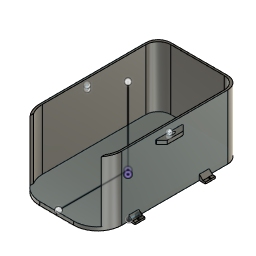
Drone_BatteryHolder v3 (Autodesk Fusion 360 design; units mm, degrees)
Autodesk Fusion 360 part; units mm, degrees
note: some values were not read from the file. Chosen so that the rebuilt part matches the saved one: which face or edge a step refers to; how an offset face is resized; which pieces of a blend or face edit are solid.
sketch "Sketch1" plane through (0, 0, 0) normal (0, 0, 1) x (1, 0, 0)
sketch "Sketch2" plane through (0, 0, 0) normal (0, 0, 1) x (1, 0, 0)
sketch "Sketch3" plane through (0, 0, 0) normal (0, 0, 1) x (1, 0, 0)
sketch "Sketch4" plane through (0, 0, 0) normal (0, 0, 1) x (1, 0, 0)
sketch "Sketch5" plane through (0, 0, 0) normal (0, 0, 1) x (1, 0, 0)
sketch "Sketch6" plane through (0, 0, 0) normal (0, 0, 1) x (1, 0, 0)
sketch "Sketch7" plane through (0, 0, 0) normal (0, 0, 1) x (1, 0, 0)
sketch "Sketch8" plane through (0, 0, 0) normal (0, 0, 1) x (1, 0, 0)
sketch "Sketch9" plane through (0, 0, 0) normal (0, 0, 1) x (1, 0, 0)
sketch "Sketch10" plane through (0, 0, 0) normal (0, 0, 1) x (1, 0, 0)
  line L0 (0, 0) -> (0, 40)
  line L1 (0, 0) -> (23, 0)
  line L2 (0, 0) -> (50, 0) construction
  line L3 (23, 0) -> (23, 40)
  line L4 (23, 40) -> (0, 40)
  line L5 (23, -40) -> (0, -40)
  line L6 (23, 0) -> (23, -40)
  line L7 (0, 0) -> (0, -40)
  line L8 (-23, 40) -> (0, 40)
  line L9 (-23, 0) -> (-23, 40)
  line L10 (0, 0) -> (-50, 0) construction
  line L11 (-23, 0) -> (-23, -40)
  line L12 (-23, -40) -> (0, -40)
  line L13 (0, 0) -> (-23, 0)
  dimension "d15" = 40
  dimension "d16" = 23
  constraint coincident L0.start L1.start
  constraint vertical L0
  constraint perpendicular L0 L1
  constraint horizontal L2
  constraint perpendicular L1 L3
  constraint symmetric L0.start L1 L2.start
  constraint symmetric L0.end L1 L5.end
  constraint symmetric L3.start L1 L6.start
  constraint symmetric L1 L3.end L5.start
  constraint symmetric L4.end L0 L8.end
  constraint symmetric L0 L1.end L9.start
  constraint symmetric L0 L1.start L2.start
  constraint symmetric L0 L2.end L10.end
  constraint symmetric L0 L3.end L8.start
  constraint symmetric L0.start L7 L1.start
  constraint symmetric L1.end L7 L9.start
  constraint symmetric L5.start L7 L11.end
  constraint symmetric L5.end L7 L12.end
  measures "d15" distance of L0.start L0.end
  measures "d16" distance of L0.start L1.end
extrude "Extrude1" add sketch "Sketch10" along normal blind 2
fillet "Fillet1" radius 7 2 edges at (23, 40, 1) (-23, 40, 1)
fillet "Fillet2" radius 13.5 2 edges at (-23, -40, 1) (23, -40, 1)
sketch "Sketch11" plane through (0, 0, 2) normal (0, 0, 1) x (-1, 0, 0)
  arc A0 (-9.5, 40) -> (-23, 26.5) centre (-9.5, 26.5) ccw
  line L0 (-23, 26.5) -> (-23, -33)
  arc A1 (-23, -33) -> (-16, -40) centre (-16, -33) ccw
  line L1 (-16, -40) -> (0, -40)
  line L2 (0, -40) -> (16, -40)
  arc A2 (16, -40) -> (23, -33) centre (16, -33) ccw
  line L3 (23, -33) -> (23, 26.5)
  arc A3 (23, 26.5) -> (9.5, 40) centre (9.5, 26.5) ccw
  line L4 (9.5, 40) -> (0, 40)
  line L5 (0, 40) -> (-9.5, 40)
  line L6 (0, 0) -> (0, -40)
  line L7 (0, 0) -> (-23, 0)
  line L8 (-23, 0) -> (-23, -33)
  line L9 (0, -40) -> (-16, -40)
  arc A4 (-23, -33) -> (-16, -40) centre (-16, -33) ccw
  line L10 (0, -39) -> (-15, -39)
  line L11 (-22, 0) -> (-22, -32)
  arc A5 (-22, -32) -> (-15, -39) centre (-15, -32) ccw
  line L12 (0, -39) -> (15, -39)
  line L13 (0, -40) -> (16, -40)
  arc A6 (16, -40) -> (23, -33) centre (16, -33) ccw
  arc A7 (15, -39) -> (22, -32) centre (15, -32) ccw
  line L14 (22, 0) -> (22, -32)
  line L15 (23, 0) -> (23, -33)
  line L16 (0, 0) -> (23, 0)
  line L17 (0, 0) -> (0, 40)
  line L18 (23, 0) -> (23, 26.5)
  line L19 (22, 0) -> (22, 26.0718)
  arc A8 (22, 26.0718) -> (20, 33) centre (9, 26.0718) ccw
  arc A9 (23, 26.5) -> (20.0018, 34.983) centre (9.5, 26.5) ccw
  line L20 (-23, 0) -> (-23, 26.5)
  line L21 (-22, 0) -> (-22, 26.0718)
  arc A10 (-20.0018, 34.983) -> (-23, 26.5) centre (-9.5, 26.5) ccw
  arc A11 (-20, 33) -> (-22, 26.0718) centre (-9, 26.0718) ccw
  line L22 (20.0018, 32.9971) -> (20.0018, 34.983)
  line L23 (-20.0018, 32.9971) -> (-20.0018, 34.983)
  dimension "d25" = 7
  dimension "d26" = 7
  constraint coincident L6.start L7.start
  constraint coincident L1.end L2.start
  constraint coincident L0 L7.end
  constraint perpendicular L0 L7
  constraint tangent L9 A4
  constraint tangent L8 A4
  constraint coincident L6 L10.start
  constraint perpendicular L6 L10
  constraint coincident L7 L11.start
  constraint perpendicular L7 L11
  constraint tangent L11 A5
  constraint tangent L10 A5
  constraint symmetric L1.end L6 L2.start
  constraint symmetric L6 L7.end L15.start
  constraint symmetric L6 A1.end L2.end
  constraint symmetric L6 L0.end A2.end
  constraint symmetric L6 A4 A6
  constraint symmetric L6 L10.start L12.start
  constraint symmetric L6 L11.start L14.start
  constraint symmetric L6 L11.end A7.end
  constraint symmetric L6 L10.end L12.end
  constraint symmetric L6 A5 A7
  constraint perpendicular L15 L16
  constraint coincident L4.end L5.start
  constraint parallel L3 L18
  constraint parallel L18 L19
  constraint tangent L19 A8
  constraint tangent L18 A9
  constraint symmetric L14.start L17 L11.start
  constraint symmetric L15.start L17 L7.end
  constraint symmetric L17 L19.end L21.end
  constraint symmetric L17 A8.end A11.start
  constraint symmetric L17 A8 A11
  constraint symmetric L17 L3.end A0.end
  constraint symmetric L17 A10.start A9.end
  constraint symmetric L17 A9 A10
  constraint coincident A8 L22.start
  constraint coincident A9 L22.end
  constraint vertical L22
  constraint symmetric L17 L22.start L23.start
  constraint symmetric L17 A9.end A10.start
  constraint coincident A0 A10.start
  measures "d25" radius of A4
  measures "d26" radius of A5
extrude "Extrude2" add sketch "Sketch11" along normal blind 34 contours A0 L0 L7 L20 L21 A10 A11 L23 | L0 A1 L1 L6 L7 L8 L9 A4 L10 L11 A5 | L3 A3 L16 L18 L19 A8 A9 L22 | L2 A2 L3 L6 L12 L13 A6 A7 L14 L15 L16
sketch "Sketch12" plane through (0, 0, 0) normal (0, 1, 0) x (1, 0, 0)
  line L0 (23, -30) -> (23, -32)
  line L1 (-23, -30) -> (-23, -32)
  constraint vertical L0
sketch "Sketch13" plane through (23, 0, 0) normal (1, 0, 0) x (0, 1, 0)
  line L0 (-26.5, 36) -> (-26.5, 0)
  line L1 (-26.5, 0) -> (33, 0)
  line L2 (33, 0) -> (33, 36)
  line L3 (33, 36) -> (-26.5, 36)
  line L4 (0, 50) -> (0, 0)
  line L5 (0, 32) -> (7.5, 32)
  line L6 (0, 32) -> (-7.5, 32)
  line L7 (7.5, 32) -> (7.5, 30)
  line L8 (7.5, 30) -> (0, 30)
  line L9 (-7.5, 32) -> (-7.5, 30)
  line L10 (-7.5, 30) -> (0, 30)
  dimension "d31" = 7.5
  constraint coincident L4.end origin
  constraint perpendicular L1 L4
  constraint coincident L4 L5.start
  constraint perpendicular L4 L5
  constraint symmetric L4 L5.start L6.start
  constraint symmetric L4 L5.end L6.end
  constraint perpendicular L5 L7
  constraint coincident L4 L8.end
  constraint perpendicular L4 L8
  constraint symmetric L4 L7.end L9.end
  constraint symmetric L4 L8.end L10.end
  measures "d31" distance of L5.start L5.end
sketch "Sketch14" plane through (-23, 0, 0) normal (-1, 0, 0) x (0, -1, 0)
  line L0 (26.5, 0) -> (26.5, 36)
  line L1 (26.5, 36) -> (-33, 36)
  line L2 (-33, 36) -> (-33, 0)
  line L3 (-33, 0) -> (26.5, 0)
  line L4 (0, 32) -> (7.5, 32)
  line L5 (7.5, 32) -> (7.5, 30)
  line L6 (7.5, 30) -> (0, 30)
  line L7 (0, 45) -> (0, 0)
  line L8 (0, 0) -> (44, 0)
  line L9 (0, 32) -> (-7.5, 32)
  line L10 (-7.5, 32) -> (-7.5, 30)
  line L11 (-7.5, 30) -> (0, 30)
  dimension "d32" = 7.5
  constraint parallel L1 L4
  constraint perpendicular L1 L5
  constraint perpendicular L5 L6
  constraint coincident L7.end L8.start
  constraint perpendicular L3 L7
  constraint perpendicular L7 L8
  constraint symmetric L4.start L7 L9.start
  constraint symmetric L4.end L7 L9.end
  constraint symmetric L5.end L7 L10.end
  constraint symmetric L6.end L7 L11.end
  measures "d32" distance of L4.start L4.end
sketch "Sketch15" plane through (0, 0, 0) normal (0, 1, 0) x (1, 0, 0)
  line L0 (0, 0) -> (0, -45)
  constraint coincident L0.start origin
  constraint vertical L0
extrude "Extrude3" add sketch "Sketch14" along normal blind 3.5 contours L4 L5 L6 L7 | L7 L9 L10 L11
extrude "Extrude4" add sketch "Sketch13" along normal blind 3.5 contours L4 L5 L7 L8 | L4 L6 L9 L10
sketch "Sketch16" plane through (0, 0, 2) normal (0, 0, 1) x (-1, 0, 0)
  line L0 (20.0018, 32.9971) -> (20.0018, 34.983)
  arc A0 (20.0018, 34.983) -> (9.5, 40) centre (9.5, 26.5) ccw
  line L1 (9.5, 40) -> (0, 40)
  line L2 (0, 40) -> (-9.5, 40)
  arc A1 (-9.5, 40) -> (-20.0018, 34.983) centre (-9.5, 26.5) ccw
  line L3 (-20.0018, 34.983) -> (-20.0018, 32.9971)
  arc A2 (-20.0018, 32.9971) -> (-22, 26.0718) centre (-9, 26.0718) ccw
  line L4 (-22, 26.0718) -> (-22, -32)
  arc A3 (-22, -32) -> (-15, -39) centre (-15, -32) ccw
  line L5 (-15, -39) -> (15, -39)
  arc A4 (15, -39) -> (22, -32) centre (15, -32) ccw
  line L6 (22, -32) -> (22, 26.0718)
  arc A5 (22, 26.0718) -> (20.0018, 32.9971) centre (9, 26.0718) ccw
chamfer "Chamfer1" distance 3 angle 45 2 edges at (-26.5, 7.5, 31) (-26.5, -7.5, 31)
chamfer "Chamfer2" distance 3 angle 45 2 edges at (26.5, 7.5, 31) (26.5, -7.5, 31)
sketch "Sketch17" plane through (0, 0, 2) normal (0, 0, 1) x (-1, 0, 0)
sketch "Sketch18" plane through (0, 0, 32) normal (0, 0, 1) x (-1, 0, 0)
  line L0 (26.5, 4.5) -> (23.5, 7.5)
  line L1 (23.5, 7.5) -> (23, 7.5)
  line L2 (23, 7.5) -> (23, -7.5)
  line L3 (23, -7.5) -> (23.5, -7.5)
  line L4 (23.5, -7.5) -> (26.5, -4.5)
  line L5 (26.5, -4.5) -> (26.5, 4.5)
  line L6 (0, 0) -> (0, -49)
  ellipse E0 centre (24.5, 0) end of major axis (24.5, -2) minor radius 0.75
  line L7 (24.5, 2) -> (24.5, -2)
  line L8 (23.75, 0) -> (25.25, 0)
  dimension "d39" = 1.5
  constraint coincident L6.start origin
  constraint vertical L6
  constraint vertical L7
  constraint coincident E0 L7.start
  constraint coincident E0 L7.end
  constraint coincident E0 L8.start
  constraint coincident E0 L8.end
extrude "Extrude5" cut sketch "Sketch18" against normal blind 2 contours E0 L7 L8 | E0 L7 L8 | E0 L7 L8 | E0 L7 L8
sketch "Sketch19" plane through (0, 0, 32) normal (0, 0, 1) x (-1, 0, 0)
  ellipse E0 centre (24.5, 0) end of major axis (24.5, -2) minor radius 0.75
  line L0 (26.5, 4.5) -> (23.5, 7.5)
  line L1 (23.5, 7.5) -> (23, 7.5)
  line L2 (23, 7.5) -> (23, -7.5)
  line L3 (23, -7.5) -> (23.5, -7.5)
  line L4 (23.5, -7.5) -> (26.5, -4.5)
  line L5 (26.5, -4.5) -> (26.5, 4.5)
  line L6 (0, 0) -> (0, -26)
  ellipse E1 centre (-24.5, 0) end of major axis (-24.5, -2) minor radius 0.75
  constraint coincident L6.start origin
  constraint vertical L6
  constraint symmetric E0 L6 E1
extrude "Extrude6" cut sketch "Sketch19" against normal blind 2 contours E1
sketch "Sketch20" plane through (-23, 0, 0) normal (-1, 0, 0) x (0, -1, 0)
  line L0 (7.5, 32) -> (7.5, 30)
  line L1 (7.5, 30) -> (-7.5, 30)
  line L2 (-7.5, 30) -> (-7.5, 32)
  line L3 (-7.5, 32) -> (7.5, 32)
  line L4 (26.5, 0) -> (26.5, 36)
  line L5 (26.5, 36) -> (-33, 36)
  line L6 (-33, 36) -> (-33, 0)
  line L7 (-33, 0) -> (26.5, 0)
  line L8 (0, 45) -> (0, 0)
  line L9 (0, 0) -> (50, 0)
  line L10 (26.5, 0) -> (22.5, 0)
  line L11 (22.5, 0) -> (22.5, 3)
  line L12 (22.5, 3) -> (17, 3)
  line L13 (17, 3) -> (17, 0)
  line L14 (-22.5, 0) -> (-22.5, 3)
  line L15 (-22.5, 3) -> (-17, 3)
  line L16 (-17, 3) -> (-17, 0)
  dimension "d44" = 4
  constraint coincident L8.end L9.start
  constraint perpendicular L7 L8
  constraint perpendicular L8 L9
  constraint coincident L4.start L7.end
  constraint perpendicular L4 L10
  constraint perpendicular L9 L11
  constraint perpendicular L11 L12
  constraint coincident L9 L13.end
  constraint perpendicular L12 L13
  constraint symmetric L8 L10.end L14.start
  constraint symmetric L8 L11.end L14.end
  constraint symmetric L8 L12.end L15.end
  constraint symmetric L8 L13.end L16.end
  measures "d44" distance of L4.start L10.end
extrude "Extrude7" add sketch "Sketch20" along normal blind 2 contours L7 L14 L15 L16 | L7 L9 L11 L12 L13
sketch "Sketch21" plane through (-23, 0, 0) normal (-1, 0, 0) x (0, -1, 0)
  line L0 (22.5, 3) -> (22.5, 0)
  line L1 (22.5, 0) -> (26.5, 0)
  line L2 (26.5, 0) -> (26.5, 36)
  line L3 (26.5, 36) -> (-33, 36)
  line L4 (-33, 36) -> (-33, 0)
  line L5 (-33, 0) -> (-22.5, 0)
  line L6 (-22.5, 0) -> (-22.5, 3)
  line L7 (-22.5, 3) -> (-17, 3)
  line L8 (-17, 3) -> (-17, 0)
  line L9 (-17, 0) -> (17, 0)
  line L10 (17, 0) -> (17, 3)
  line L11 (17, 3) -> (22.5, 3)
  line L12 (7.5, 32) -> (7.5, 30)
  line L13 (7.5, 30) -> (-7.5, 30)
  line L14 (-7.5, 30) -> (-7.5, 32)
  line L15 (-7.5, 32) -> (7.5, 32)
sketch "Sketch22" plane through (23, 0, 0) normal (1, 0, 0) x (0, 1, 0)
  line L0 (7.5, 32) -> (7.5, 30)
  line L1 (7.5, 30) -> (-7.5, 30)
  line L2 (-7.5, 30) -> (-7.5, 32)
  line L3 (-7.5, 32) -> (7.5, 32)
  line L4 (-26.5, 36) -> (-26.5, 0)
  line L5 (-26.5, 0) -> (33, 0)
  line L6 (33, 0) -> (33, 36)
  line L7 (33, 36) -> (-26.5, 36)
  line L8 (0, 45) -> (0, 0)
  line L9 (0, 0) -> (50, 0)
  line L10 (-26.5, 0) -> (-22.5, 0)
  line L11 (-22.5, 0) -> (-22.5, 3)
  line L12 (-22.5, 3) -> (-18.5, 3)
  line L13 (-18.5, 3) -> (-18.5, 0)
  line L14 (22.5, 0) -> (22.5, 3)
  line L15 (22.5, 3) -> (18.5, 3)
  line L16 (18.5, 3) -> (18.5, 0)
  dimension "d47" = 4
  dimension "d48" = 3
  dimension "d49" = 4
  constraint coincident L8.end L9.start
  constraint perpendicular L5 L8
  constraint perpendicular L8 L9
  constraint coincident L4.end L5.start
  constraint perpendicular L4 L10
  constraint perpendicular L10 L11
  constraint perpendicular L11 L12
  constraint coincident L5 L13.end
  constraint perpendicular L5 L13
  constraint symmetric L8 L10.end L14.start
  constraint symmetric L8 L11.end L14.end
  constraint symmetric L8 L12.end L15.end
  constraint symmetric L8 L13.end L16.end
  measures "d47" distance of L4.end L10.end
  measures "d48" distance of L10.end L11.end
  measures "d49" distance of L11.end L12.end
extrude "Extrude8" add sketch "Sketch22" along normal blind 2 contours L5 L11 L12 L13 | L5 L9 L14 L15 L16
delete_face "DeleteFace1" 5 faces at (24.3333, -22.5, 1.6667) (23.6667, -21.1667, 3) (24.3333, -18.5, 1.6667) (23.6667, -21.1667, 0) (25, -19.8333, 1)
delete_face "DeleteFace2" 1 faces at (23.6667, 21.1667, 3)
sketch "Sketch23" plane through (23, 0, 0) normal (1, 0, 0) x (0, 1, 0)
  line L0 (7.5, 32) -> (7.5, 30)
  line L1 (7.5, 30) -> (-7.5, 30)
  line L2 (-7.5, 30) -> (-7.5, 32)
  line L3 (-7.5, 32) -> (7.5, 32)
  line L4 (33, 36) -> (-26.5, 36)
  line L5 (-26.5, 36) -> (-26.5, 0)
  line L6 (-26.5, 0) -> (33, 0)
  line L7 (33, 0) -> (33, 36)
  line L8 (0, 0) -> (0, 45)
  line L9 (0, 0) -> (45, 0)
  line L10 (-26.5, 0) -> (-22.5, 0)
  line L11 (-22.5, 0) -> (-17, 0)
  line L12 (-22.5, 0) -> (-22.5, 3)
  line L13 (-22.5, 3) -> (-17, 3)
  line L14 (-17, 3) -> (-17, 0)
  line L15 (22.5, 0) -> (22.5, 3)
  line L16 (22.5, 3) -> (17, 3)
  line L17 (17, 3) -> (17, 0)
  dimension "d52" = 4
  constraint coincident L8.start L9.start
  constraint perpendicular L4 L8
  constraint perpendicular L8 L9
  constraint coincident L5.end L6.start
  constraint coincident L6 L10.end
  constraint coincident L6 L11.end
  constraint perpendicular L11 L12
  constraint perpendicular L12 L13
  constraint perpendicular L6 L14
  constraint symmetric L8 L10.end L15.start
  constraint symmetric L8 L11.end L17.end
  constraint symmetric L8 L12.end L15.end
  constraint symmetric L8 L13.end L16.end
  measures "d52" distance of L5.end L10.end
extrude "Extrude9" add sketch "Sketch23" along normal blind 2 contours L6 L11 L12 L13 L14 | L6 L9 L15 L16 L17
chamfer "Chamfer3" distance 2 angle 45 4 edges at (25, -19.75, 3) (25, 19.75, 3) (-25, -19.75, 3) (-25, 19.75, 3)
sketch "Sketch24" plane through (23, 0, 0) normal (1, 0, 0) x (0, 1, 0)
  line L0 (22.5, 3) -> (22.5, 0)
  line L1 (22.5, 0) -> (33, 0)
  line L2 (33, 0) -> (33, 36)
  line L3 (33, 36) -> (-26.5, 36)
  line L4 (-26.5, 36) -> (-26.5, 0)
  line L5 (-26.5, 0) -> (-22.5, 0)
  line L6 (-22.5, 0) -> (-22.5, 3)
  line L7 (-22.5, 3) -> (-17, 3)
  line L8 (-17, 3) -> (-17, 0)
  line L9 (-17, 0) -> (17, 0)
  line L10 (17, 0) -> (17, 3)
  line L11 (17, 3) -> (22.5, 3)
  line L12 (7.5, 32) -> (7.5, 30)
  line L13 (7.5, 30) -> (-7.5, 30)
  line L14 (-7.5, 30) -> (-7.5, 32)
  line L15 (-7.5, 32) -> (7.5, 32)
  line L16 (-22.5, 0.9094) -> (-17, 0.9094)
  line L17 (-17, 0.9094) -> (-17, 0)
  line L18 (-17, 0) -> (-22.5, 0)
  line L19 (-22.5, 0) -> (-22.5, 0.9094)
  constraint horizontal L16
  constraint vertical L17
  constraint horizontal L18
  constraint vertical L19
  constraint coincident L8.end L9.start
  constraint coincident L6 L16.start
sketch "Sketch25" plane through (0, 0, 2) normal (0, 0, 1) x (-1, 0, 0)
sketch "Sketch26" plane through (0, 0, 2) normal (0, 0, 1) x (-1, 0, 0)
sketch "Sketch27" plane through (0, 0, 2) normal (0, 0, 1) x (-1, 0, 0)
sketch "Sketch28" plane through (0, 0, 0) normal (0, 0, 1) x (1, 0, 0)
sketch "Sketch29" plane through (0, 0, 0) normal (0, 0, 1) x (1, 0, 0)
sketch "Sketch30" plane through (0, 0, 0) normal (0, 0, 1) x (1, 0, 0)
  line L0 (0, -50) -> (0, 45)
  line L1 (-35, 0) -> (39, 0)
  line L2 (-25, -22.5) -> (-26.5, -22.5)
  line L3 (-26.5, -22.5) -> (-26.5, -17)
  line L4 (-26.5, -17) -> (-25, -17)
  line L5 (-25, -17) -> (-25, -22.5)
  line L6 (-26.5, 22.5) -> (-26.5, 17)
  line L7 (-25, 22.5) -> (-26.5, 22.5)
  line L8 (-25, 17) -> (-25, 22.5)
  line L9 (-26.5, 17) -> (-25, 17)
  constraint vertical L0
  constraint horizontal L1
  constraint horizontal L2
  constraint vertical L3
  constraint horizontal L4
  constraint vertical L5
  constraint symmetric L1 L2.start L7.start
  constraint symmetric L1 L2.end L6.start
  constraint symmetric L1 L3.end L6.end
  constraint symmetric L1 L4.end L8.start
extrude "Extrude10" add sketch "Sketch30" along normal blind 1
sketch "Sketch31" plane through (0, 0, 0) normal (0, 0, 1) x (1, 0, 0)
  line L0 (0, 0) -> (40, 0)
  line L1 (25, -22.5) -> (26.5, -22.5)
  line L2 (26.5, -22.5) -> (26.5, -17)
  line L3 (26.5, -17) -> (25, -17)
  line L4 (25, -17) -> (25, -22.5)
  line L5 (25, 22.5) -> (26.5, 22.5)
  line L6 (25, 17) -> (25, 22.5)
  line L7 (26.5, 22.5) -> (26.5, 17)
  line L8 (26.5, 17) -> (25, 17)
  constraint coincident L0.start origin
  constraint horizontal L0
  constraint horizontal L1
  constraint vertical L2
  constraint horizontal L3
  constraint vertical L4
  constraint symmetric L0 L1.start L5.start
  constraint symmetric L0 L1.end L5.end
  constraint symmetric L0 L2.end L7.end
  constraint symmetric L0 L3.end L6.start
extrude "Extrude11" add sketch "Sketch31" along normal blind 1
sketch "Sketch32" plane through (0, 0, 2) normal (0, 0, 1) x (-1, 0, 0)
sketch "Sketch33" plane through (0, 0, 0) normal (0, 0, 1) x (1, 0, 0)
sketch "Sketch34" plane through (0, 0, 2) normal (0, 0, 1) x (-1, 0, 0)
  line L0 (0, 0) -> (0, 39)
  constraint coincident L0.start origin
  constraint vertical L0
sketch "Sketch35" plane through (0, 0, 2) normal (0, 0, 1) x (-1, 0, 0)
  line L0 (25.7, 20) -> (-25.7, 20)
  line L1 (-25.7, 20) -> (-25.7, -20)
  line L2 (-25.7, -20) -> (25.7, -20)
  line L3 (25.7, -20) -> (25.7, 20)
  line L4 (25.7, 20) -> (-25.7, -20) construction
  line L5 (-25.7, 20) -> (25.7, -20) construction
  point P0 (25.7, 20)
  point P1 (25.7, -20)
  point P2 (-25.7, -20)
  point P3 (-25.7, 20)
  constraint horizontal L0
  constraint perpendicular L0 L1
  constraint parallel L0 L2
  constraint parallel L1 L3
  constraint coincident L4 origin
  constraint coincident L5 origin
  constraint coincident P0 L0.start
  constraint coincident P1 L2.end
  constraint coincident P2 L1.end
  constraint coincident P3 L0.end
hole "Hole1" at (-25.7, -20, 2) at (-25.7, 20, 2) at (25.7, 20, 2) at (25.7, -20, 2) direction (0, 0, -1) diameter 0.769 depth 2 tip angle 118
thread "Thread1" "ISO Metric profile 1.0 M1x0.2 6H" major diameter 1.0461 minor diameter 0.821 pitch 0.2 angle 60 resizes the face on face at (-25.9005, -20.3281, 0.6667) on face at (-25.9005, 19.6719, 0.6667) on face at (25.4995, 19.6719, 0.6667) on face at (25.4995, -20.3281, 0.6667)
